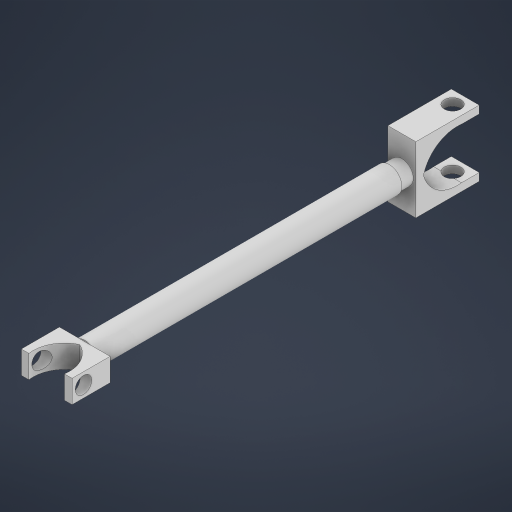
# Autodesk Inventor part: Part1
Saved by Autodesk Inventor 2023 (Build 270158030, 158C)
## iProperties
Created: 2023-02-03
Part Number: Part1
Material: Generic
Document SubType Name: Modeling
Designer: Monster
Density: 1 g/cm^3
Appearance: Default
Author: Monster
Autodesk Inventor part; units mm, degrees
ref_plane "YZ Plane" through (0, 0, 0) normal (1, 0, 0) x (0, 1, 0)
ref_plane "XZ Plane" through (0, 0, 0) normal (0, 1, 0) x (-1, 0, 0)
ref_plane "XY Plane" through (0, 0, 0) normal (0, 0, 1) x (1, 0, 0)
sketch "Sketch1" plane through (0, 0, 0) normal (0, 0, 1) x (1, 0, 0)
  circle A0 centre (0, 0) radius 5
  dimension "d0" = 10
  constraints: 1 centre point, 1 coincident
  measures "d0" diameter of A0
extrude "Extrusion1" add sketch "Sketch1" against normal blind 120
sketch "Sketch2" plane through (0, 0, -120) normal (0, 0, -1) x (-1, 0, 0)
  circle A0 centre (0, 0) radius 4.5
  dimension "d3" = 9
  constraints: 1 centre point, 1 coincident
  measures "d3" diameter of A0
extrude "Extrusion2" add sketch "Sketch2" along normal blind 5
sketch "Sketch3" plane through (0, 0, 0) normal (0, 0, 1) x (1, 0, 0)
  circle A0 centre (0, 0) radius 5 projected
  line L0 (0, 0) -> (10, 0)
  line L1 (10, 0) -> (-10, 0)
  line L2 (0, 0) -> (0, 4.5)
  line L3 (0, 4.5) -> (0, -4.5)
  line L4 (0, -4.5) -> (-10, -4.5)
  line L5 (-10, -4.5) -> (-10, 0)
  line L6 (-10, 0) -> (-10, 4.5)
  line L7 (-10, 4.5) -> (0, 4.5)
  line L8 (0, 4.5) -> (10, 4.5)
  line L9 (10, 4.5) -> (10, -4.5)
  line L10 (10, -4.5) -> (0, -4.5)
  dimension "d8" = 4.5
  dimension "d53" = 4.5
  dimension "d56" = 20
  dimension "d57" = 10
  dimension "d58" = 10
  constraints: 22 end point, 5 perpendicular, 5 point on line, 1 horizontal, 1 vertical
  measures "d8" distance of L0.start L2.end
  measures "d53" distance between parallel lines of L4 L1
  measures "d56" distance between parallel lines of L9 L5
  measures "d57" distance between parallel lines of L3 L5
  measures "d58" distance between parallel lines of L3 L9
extrude "Extrusion3" add sketch "Sketch3" along normal blind 15 contours L0 L2 L8 A0 | L0 L9 L10 A0 | A0 L10 L3 L0 | A0 L8 L9 L0 | L3 L4 A0 L1 | L1 A0 L7 L2 | A0 L1 L6 L7 | L4 L5 L1 A0
sketch "Sketch4" plane through (-10, -4.5, 0) normal (0, -1, 0) x (1, 0, 0)
  line L0 (0, 0) -> (7.8206, 0) projected
  line L1 (12.1794, 0) -> (7.8206, 0) projected
  line L2 (12.1794, 0) -> (20, 0) projected
  line L3 (20, 0) -> (20, 15) projected
  line L4 (0, 15) -> (20, 15) projected
  line L5 (0, 0) -> (0, 15) projected
  line L6 (10, 0) -> (10, 2)
  line L7 (0, 15) -> (20, 15) projected
  line L8 (0, 15) -> (3, 15)
  line L9 (20, 15) -> (17, 15)
  arc A0 (3, 15) -> (10, 2) centre (15.2365, 13.2043) ccw
  line L10 (10, 2) -> (10, 15)
  line L11 (4.3472, 7.3408) -> (0, 7.3408)
  line L12 (0, 0) -> (0, 15) projected
  line L13 (4.3472, 7.3408) -> (4.3472, 0)
  line L14 (15.6528, 7.3408) -> (20, 7.3408)
  line L15 (15.6528, 7.3408) -> (15.6528, 0)
  arc A1 (10, 2) -> (17, 15) centre (4.7635, 13.2043) ccw
  dimension "d12" = 2
  dimension "d13" = 3
  dimension "d14" = 3
  constraints: 16 end point, 6 point on circle, 4 point on line, 3 symmetric about line, 2 centre point, 2 perpendicular, 1 midpoint, 1 vertical
  measures "d12" distance of L6.start L6.end
  measures "d13" distance of L4.start L8.end
  measures "d14" distance of L3.end L9.end
extrude "Extrusion4" cut sketch "Sketch4" against normal blind 15 contours A0 L4 L10 | L10 L4 A1
sketch "Sketch5" plane through (10, -4.5, 0) normal (1, 0, 0) x (0, 0, -1)
  line L0 (0, 0) -> (0, 9) projected
  line L1 (0, 9) -> (-15, 9) projected
  line L2 (-15, 0) -> (-15, 9) projected
  line L3 (0, 0) -> (-15, 0) projected
  line L4 (-15, 0) -> (-15, 9) projected
  line L5 (-15, 4.5) -> (-10.5, 4.5)
  line L6 (0, 9) -> (0, 0) projected
  circle A0 centre (-10.5, 4.5) radius 3.25
  point P0 (0, 4.5)
  dimension "d19" = 4.5
  dimension "d55" = 6.5
  constraints: 2 end point, 1 centre point, 1 coincident, 1 midpoint, 1 perpendicular
  measures "d19" distance of L5.start L5.end
  measures "d55" diameter of A0
extrude "Extrusion5" cut sketch "Sketch5" against normal blind 37.25 contours A0
sketch "Sketch6" plane through (0, 0, -125) normal (0, 0, -1) x (-1, 0, 0)
  circle A0 centre (0, 0) radius 4.5 projected
  line L0 (0, 0) -> (0, 13)
  line L1 (0, -4.5) -> (0, 4.5) projected
  line L2 (0, 13) -> (0, -13)
  line L3 (0, -13) -> (-5.5, -13)
  line L4 (-5.5, -13) -> (5.5, -13)
  line L5 (5.5, -13) -> (5.5, 13)
  line L6 (5.5, 13) -> (-5.5, 13)
  line L7 (-5.5, 13) -> (-5.5, -13)
  dimension "d23" = 13
  dimension "d24" = 26
  dimension "d25" = 5.5
  dimension "d26" = 11
  constraints: 14 end point, 4 perpendicular, 1 collinear, 1 horizontal, 1 point on line
  measures "d23" distance of L0.start L0.end
  measures "d24" distance of L0.end L2.end
  measures "d25" distance of L2.end L3.end
  measures "d26" distance of L3.end L4.end
extrude "Extrusion6" add sketch "Sketch6" along normal blind 25
sketch "Sketch7" plane through (5.5, -13, -125) normal (1, 0, 0) x (0, 0, -1)
  line L0 (0, 26) -> (0, 0) projected
  line L1 (0, 0) -> (25, 0) projected
  line L2 (25, 26) -> (25, 0) projected
  line L3 (0, 26) -> (25, 26) projected
  line L4 (25, 26) -> (25, 0) projected
  line L5 (25, 26) -> (25, 23)
  line L6 (25, 0) -> (25, 3)
  line L7 (25, 23) -> (18, 23)
  line L8 (0, 8.5) -> (0, 17.5) projected
  line L9 (0, 13) -> (3, 13)
  arc A0 (18, 23) -> (3, 13) centre (16.2622, 9.3566) ccw
  line L10 (25, 3) -> (18, 3)
  line L11 (18, 3) -> (18, 23)
  arc A1 (3, 13) -> (18, 3) centre (16.3321, 16.7481) ccw
  point P0 (-125, 13)
  dimension "d29" = 3
  dimension "d30" = 3
  dimension "d32" = 7
  dimension "d33" = 3
  constraints: 12 end point, 4 point on circle, 3 horizontal, 2 centre point, 2 point on line, 1 midpoint, 1 perpendicular
  measures "d29" distance of L2.start L5.end
  measures "d30" distance of L1.end L6.end
  measures "d32" distance of L5.end L7.end
  measures "d33" distance of L9.start L9.end
extrude "Extrusion7" cut sketch "Sketch7" against normal blind 25 contours L2 L10 L11 L7 | A0 L11 A1
sketch "Sketch8" plane through (-5.5, 13, -125) normal (0, 1, 0) x (1, 0, 0)
  line L0 (0, 0) -> (11, 0) projected
  line L1 (11, 0) -> (11, 25) projected
  line L2 (0, 25) -> (11, 25) projected
  line L3 (0, 0) -> (0, 25) projected
  line L4 (5.5, 25) -> (5.5, 20)
  circle A0 centre (5.5, 20) radius 3.25
  line L5 (2.25, 20) -> (0, 20)
  line L6 (0, 18) -> (0, 25) projected
  line L7 (8.75, 20) -> (11, 20)
  line L8 (11, 25) -> (11, 18) projected
  point P0 (5.5, -125)
  dimension "d36" = 5
  dimension "d54" = 6.5
  constraints: 6 end point, 4 point on line, 2 point on circle, 1 centre point, 1 coincident, 1 midpoint, 1 perpendicular, 1 vertical
  measures "d36" distance of L4.start L4.end
  measures "d54" diameter of A0
extrude "Extrusion8" cut sketch "Sketch8" against normal blind 30 contours A0
body "Solid1"
